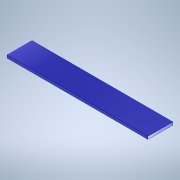
# Autodesk Inventor part: Antenna
Saved by Autodesk Inventor 2020 (Build 240168000, 168)
## iProperties
Created: 2021-10-31
Part Number: Antenna
Material: 一般
Document SubType Name: Modeling
Designer: Masato Kubotera
Density: 1 g/cm^3
Appearance: 青 - 壁塗料 - 光沢
Description: 既製品
Author: Masato Kubotera
Comments: https://www.amazon.co.jp/%E9%AB%98%E6%80%A7%E8%83%BD5dBi-2-4GHz-802-11a-%E7%84%A1%E7%B7%9ALAN%E3%82%AB%E3%83%BC%E3%83%89-Bluetooth%E3%83%A2%E3%82%B8%E3%83%A5%E3%83%BC%E3%83%AB%E7%94%A8%E3%82%A2%E3%83%B3%E3%83%86%E3%83%8A/dp/B06ZZC4WQG/ref=sr_1_15?__mk_ja_JP=%E3%82%AB%E3%82%BF%E3%82%AB%E3%83%8A&keywords=Wi-Fi+%E3%82%A2%E3%83%B3%E3%83%86%E3%83%8A&sr=8-15
Autodesk Inventor part; units mm, degrees
ref_plane "YZ Plane" through (0, 0, 0) normal (1, 0, 0) x (0, 1, 0)
ref_plane "XZ Plane" through (0, 0, 0) normal (0, 1, 0) x (-1, 0, 0)
ref_plane "XY Plane" through (0, 0, 0) normal (0, 0, 1) x (1, 0, 0)
sketch "スケッチ1" plane through (0, 0, 0) normal (0, 0, 1) x (1, 0, 0)
  line L0 (-25.5, 4.5) -> (25.5, 4.5)
  line L1 (25.5, 4.5) -> (25.5, -4.5)
  line L2 (25.5, -4.5) -> (-25.5, -4.5)
  line L3 (-25.5, -4.5) -> (-25.5, 4.5)
  line L4 (-25.5, 4.5) -> (25.5, -4.5) construction
  line L5 (25.5, 4.5) -> (-25.5, -4.5) construction
  point P0 (0, 0)
  dimension "d0" = 51
  dimension "d1" = 9
  constraints: 12 end point, 2 midpoint, 2 parallel, 1 horizontal, 1 perpendicular
  measures "d0" distance of L1.end L2.end
  measures "d1" distance of L0.end L1.end
extrude "押し出し1" add sketch "スケッチ1" along normal blind 1
